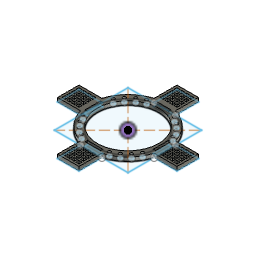
drone_option3 (Autodesk Fusion 360 design; units mm, degrees)
Autodesk Fusion 360 part; units mm, degrees
sketch "Droneframe_main_extrude" plane through (0, 0, 0) normal (0, 0, 1) x (1, 0, 0)
  circle A0 centre (0, 0) radius 50
  circle A1 centre (0, 0) radius 40
  line L0 (48, -48) -> (-48, -48)
  line L1 (-48, -48) -> (-48, 48)
  line L2 (-48, 48) -> (48, 48)
  line L3 (48, 48) -> (48, -48)
  line L4 (48, -48) -> (-48, 48) construction
  line L5 (-48, -48) -> (48, 48) construction
  line L6 (-9.9355, 46) -> (10.0645, 46)
  line L7 (10.0645, 46) -> (10.0645, 43)
  line L8 (10.0645, 43) -> (-9.9355, 43)
  line L9 (-9.9355, 43) -> (-9.9355, 46)
  line L10 (46, -9.9355) -> (46, 10.0645)
  line L11 (43, -9.9355) -> (46, -9.9355)
  line L12 (43, 10.0645) -> (43, -9.9355)
  line L13 (46, 10.0645) -> (43, 10.0645)
  line L14 (-46, 9.9355) -> (-46, -10.0645)
  line L15 (-43, 9.9355) -> (-46, 9.9355)
  line L16 (-43, -10.0645) -> (-43, 9.9355)
  line L17 (-46, -10.0645) -> (-43, -10.0645)
  line L18 (-10.0645, -43) -> (9.9355, -43)
  line L19 (-10.0645, -46) -> (-10.0645, -43)
  line L20 (9.9355, -46) -> (-10.0645, -46)
  line L21 (9.9355, -43) -> (9.9355, -46)
  line L22 (-48, -14) -> (-78, -14)
  line L23 (-78, -14) -> (-78, 14)
  line L24 (-78, 14) -> (-48, 14)
  line L25 (-48, 14) -> (-48, -14)
  line L26 (14, -78) -> (14, -48)
  line L27 (-14, -78) -> (14, -78)
  line L28 (-14, -48) -> (-14, -78)
  line L29 (-14, 78) -> (-14, 48)
  line L30 (14, 78) -> (-14, 78)
  line L31 (14, 48) -> (14, 78)
  line L32 (48, 14) -> (78, 14)
  line L33 (78, 14) -> (78, -14)
  line L34 (78, -14) -> (48, -14)
  circle A2 centre (-39.9321, 20.7467) radius 2
  circle A3 centre (-34.0712, 29.3965) radius 2
  circle A4 centre (-26.3735, 36.4615) radius 2
  circle A5 centre (-17.254, 41.5608) radius 2
  circle A6 centre (-20.7467, -39.9321) radius 2
  circle A7 centre (-29.3965, -34.0712) radius 2
  circle A8 centre (-36.4615, -26.3735) radius 2
  circle A9 centre (-41.5608, -17.254) radius 2
  circle A10 centre (39.9321, -20.7467) radius 2
  circle A11 centre (34.0712, -29.3965) radius 2
  circle A12 centre (26.3735, -36.4615) radius 2
  circle A13 centre (17.254, -41.5608) radius 2
  circle A14 centre (20.7467, 39.9321) radius 2
  circle A15 centre (29.3965, 34.0712) radius 2
  circle A16 centre (36.4615, 26.3735) radius 2
  circle A17 centre (41.5608, 17.254) radius 2
  dimension "d1" = 100
  dimension "d2" = 80
  dimension "d3" = 20
  dimension "d4" = 3
  dimension "d5" = 43
  dimension "d6" = 30
  dimension "d11" = 4
  constraint coincident A0.centre A1.centre
  constraint horizontal L0
  constraint perpendicular L0 L1
  constraint parallel L0 L2
  constraint parallel L1 L3
  constraint coincident L4 A0.centre
  constraint coincident L5 A0.centre
  constraint horizontal L6
  constraint vertical L7
  constraint horizontal L8
  constraint vertical L9
  constraint symmetric L5 L6.start L10.start
  constraint symmetric L5 L6.end L10.end
  constraint symmetric L5 L7.end L12.start
  constraint symmetric L5 L8.end L11.start
  constraint symmetric L4 L6.start L14.start
  constraint symmetric L4 L6.end L14.end
  constraint symmetric L4 L7.end L16.start
  constraint symmetric L4 L8.end L15.start
  constraint symmetric L4 L10.start L20.start
  constraint symmetric L4 L10.end L19.start
  constraint symmetric L4 L11.start L18.end
  constraint symmetric L4 L12.start L18.start
  constraint horizontal L22
  constraint vertical L23
  constraint horizontal L24
  constraint vertical L25
  constraint coincident A0 L22.start
  constraint coincident A0 L24.end
  constraint coincident L1 L24.end
  constraint symmetric L5 L22.start L28.start
  constraint symmetric L5 L22.end L27.start
  constraint symmetric L5 L23.end L26.start
  constraint symmetric L5 L24.end L26.end
  constraint symmetric L4 L22.start L31.start
  constraint symmetric L4 L22.end L30.start
  constraint symmetric L4 L23.end L29.start
  constraint symmetric L4 L24.end L29.end
  constraint symmetric L4 L26.start L33.end
  constraint symmetric L4 L26.end L34.end
  constraint symmetric L4 L27.start L32.end
  constraint symmetric L4 L28.start L32.start
  measures "d1" diameter of A0
  measures "d2" diameter of A1
  measures "d3" distance of L6.start L6.end
  measures "d4" distance of L6.start L8.end
  measures "d5" distance of A0.centre L8
  measures "d6" distance of L23.end L24.end
  measures "d11" diameter of A2
extrude "Extrude2" add sketch "Droneframe_main_extrude" along normal blind 5 contours A0 L3 | A0 L32 L33 L34 | A0 L0 L1 L2 L3 L25 | A0 L2 | A0 L29 L30 L31 | A0 L26 L27 L28 | A0 L0 | A0 L1 L25 | A0 L22 L23 L24
sketch "fin_sqaure_cuts" plane through (0, 0, 5) normal (0, 0, 1) x (-1, 0, 0)
  circle A0 centre (36.4615, 26.3735) radius 2
  circle A1 centre (39.9321, -20.7467) radius 2
  circle A2 centre (41.5608, 17.254) radius 2
  circle A3 centre (29.3965, 34.0712) radius 2
  circle A4 centre (20.7467, 39.9321) radius 2
  circle A5 centre (17.254, -41.5608) radius 2
  circle A6 centre (26.3735, -36.4615) radius 2
  circle A7 centre (34.0712, -29.3965) radius 2
  circle A8 centre (0, 0) radius 40
  line L0 (-10.0645, -43) -> (9.9355, -43)
  line L1 (9.9355, -43) -> (9.9355, -46)
  line L2 (9.9355, -46) -> (-10.0645, -46)
  line L3 (-10.0645, -46) -> (-10.0645, -43)
  line L4 (-43, -10.0645) -> (-46, -10.0645)
  line L5 (-46, -10.0645) -> (-46, 9.9355)
  line L6 (-46, 9.9355) -> (-43, 9.9355)
  line L7 (-43, 9.9355) -> (-43, -10.0645)
  circle A9 centre (-41.5608, -17.254) radius 2
  circle A10 centre (-36.4615, -26.3735) radius 2
  circle A11 centre (-29.3965, -34.0712) radius 2
  circle A12 centre (-20.7467, -39.9321) radius 2
  circle A13 centre (-17.254, 41.5608) radius 2
  circle A14 centre (-26.3735, 36.4615) radius 2
  circle A15 centre (-34.0712, 29.3965) radius 2
  circle A16 centre (-39.9321, 20.7467) radius 2
  line L8 (10.0645, 43) -> (-9.9355, 43)
  line L9 (-9.9355, 43) -> (-9.9355, 46)
  line L10 (-9.9355, 46) -> (10.0645, 46)
  line L11 (10.0645, 46) -> (10.0645, 43)
  line L12 (43, 10.0645) -> (46, 10.0645)
  line L13 (46, 10.0645) -> (46, -9.9355)
  line L14 (46, -9.9355) -> (43, -9.9355)
  line L15 (43, -9.9355) -> (43, 10.0645)
  arc A17 (-48, -14) -> (-14, -48) centre (0, 0) ccw
  line L16 (-14, -48) -> (-14, -78)
  line L17 (-14, -78) -> (14, -78)
  line L18 (14, -78) -> (14, -48)
  arc A18 (14, -48) -> (48, -14) centre (0, 0) ccw
  line L19 (48, -14) -> (78, -14)
  line L20 (78, -14) -> (78, 14)
  line L21 (78, 14) -> (48, 14)
  arc A19 (48, 14) -> (14, 48) centre (0, 0) ccw
  line L22 (14, 48) -> (14, 78)
  line L23 (14, 78) -> (-14, 78)
  line L24 (-14, 78) -> (-14, 48)
  arc A20 (-14, 48) -> (-48, 14) centre (0, 0) ccw
  line L25 (-48, 14) -> (-78, 14)
  line L26 (-78, 14) -> (-78, -14)
  line L27 (-78, -14) -> (-48, -14)
  line L28 (75, -11) -> (71, -11)
  line L29 (71, -11) -> (71, -7)
  line L30 (71, -7) -> (75, -7)
  line L31 (75, -7) -> (75, -11)
  line L32 (78, -14) -> (48, -14)
  line L33 (78, 14) -> (78, -14)
  line L34 (69, -11) -> (65, -11)
  line L35 (69, -7) -> (69, -11)
  line L36 (65, -11) -> (65, -7)
  line L37 (65, -7) -> (69, -7)
  line L38 (63, -11) -> (59, -11)
  line L39 (63, -7) -> (63, -11)
  line L40 (59, -11) -> (59, -7)
  line L41 (59, -7) -> (63, -7)
  line L42 (57, -11) -> (53, -11)
  line L43 (57, -7) -> (57, -11)
  line L44 (53, -11) -> (53, -7)
  line L45 (53, -7) -> (57, -7)
  line L46 (75, -5) -> (71, -5)
  line L47 (75, -1) -> (75, -5)
  line L48 (71, -5) -> (71, -1)
  line L49 (71, -1) -> (75, -1)
  line L50 (69, -5) -> (65, -5)
  line L51 (69, -1) -> (69, -5)
  line L52 (65, -5) -> (65, -1)
  line L53 (65, -1) -> (69, -1)
  line L54 (63, -5) -> (59, -5)
  line L55 (63, -1) -> (63, -5)
  line L56 (59, -5) -> (59, -1)
  line L57 (59, -1) -> (63, -1)
  line L58 (57, -5) -> (53, -5)
  line L59 (57, -1) -> (57, -5)
  line L60 (53, -5) -> (53, -1)
  line L61 (53, -1) -> (57, -1)
  line L62 (75, 1) -> (71, 1)
  line L63 (75, 5) -> (75, 1)
  line L64 (71, 1) -> (71, 5)
  line L65 (71, 5) -> (75, 5)
  line L66 (69, 1) -> (65, 1)
  line L67 (69, 5) -> (69, 1)
  line L68 (65, 1) -> (65, 5)
  line L69 (65, 5) -> (69, 5)
  line L70 (63, 1) -> (59, 1)
  line L71 (63, 5) -> (63, 1)
  line L72 (59, 1) -> (59, 5)
  line L73 (59, 5) -> (63, 5)
  line L74 (57, 1) -> (53, 1)
  line L75 (57, 5) -> (57, 1)
  line L76 (53, 1) -> (53, 5)
  line L77 (53, 5) -> (57, 5)
  line L78 (75, 7) -> (71, 7)
  line L79 (75, 11) -> (75, 7)
  line L80 (71, 7) -> (71, 11)
  line L81 (71, 11) -> (75, 11)
  line L82 (69, 7) -> (65, 7)
  line L83 (69, 11) -> (69, 7)
  line L84 (65, 7) -> (65, 11)
  line L85 (65, 11) -> (69, 11)
  line L86 (63, 7) -> (59, 7)
  line L87 (63, 11) -> (63, 7)
  line L88 (59, 7) -> (59, 11)
  line L89 (59, 11) -> (63, 11)
  line L90 (57, 7) -> (53, 7)
  line L91 (57, 11) -> (57, 7)
  line L92 (53, 7) -> (53, 11)
  line L93 (53, 11) -> (57, 11)
  dimension "d22" = 4
  dimension "d23" = 4
  dimension "d24" = 3
  dimension "d25" = 3
  dimension "d28" = -18
  dimension "d29" = 18
  constraint horizontal L28
  constraint vertical L29
  constraint horizontal L30
  constraint vertical L31
  measures "d22" distance of L28.start L28.end
  measures "d23" distance of L28.start L30.end
  measures "d24" distance of L28 L32
  measures "d25" distance of L31 L33
extrude "Extrude3" cut sketch "fin_sqaure_cuts" against normal blind 5 contours L28 L29 L30 L31 | L34 L35 L36 L37 | L38 L39 L40 L41 | L42 L43 L44 L45 | L46 L47 L48 L49 | L50 L51 L52 L53 | L54 L55 L56 L57 | L58 L59 L60 L61 | L62 L63 L64 L65 | L66 L67 L68 L69 | L70 L71 L72 L73 | L74 L75 L76 L77 | L78 L79 L80 L81 | L82 L83 L84 L85 | L86 L87 L88 L89 | L90 L91 L92 L93
pattern_circular "C-Pattern1" count 4 over 360 about axis through (0, 0, 1.75) along (0, 0, 1) of "Extrude3"
